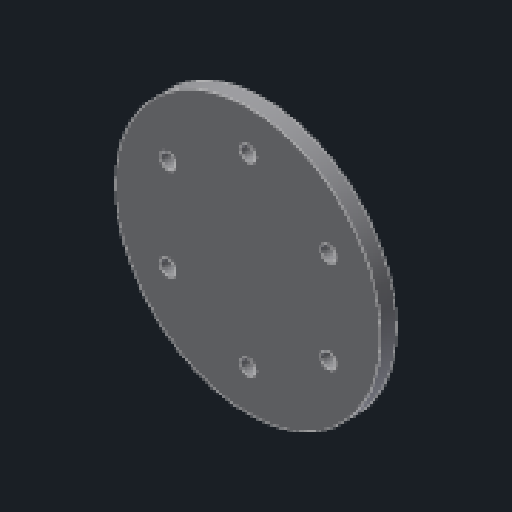
# Autodesk Inventor part: WheelSproketHub
Saved by Autodesk Inventor 2025.2 (Build 292293000, 293)
## iProperties
Created: 2025-10-03
Part Number: WheelSproketHub
Material: Generic
Document SubType Name: Sheet Metal
Designer: valer
Density: 1 g/cm^3
Appearance: Default
Sheet Metal Rule: Default
Author: valer
Autodesk Inventor part; units mm, degrees
ref_plane "YZ Plane" through (0, 0, 0) normal (1, 0, 0) x (0, 1, 0)
ref_plane "XZ Plane" through (0, 0, 0) normal (0, 1, 0) x (-1, 0, 0)
ref_plane "XY Plane" through (0, 0, 0) normal (0, 0, 1) x (1, 0, 0)
sketch "Base" plane through (0, 0, 0) normal (0, 0, 1) x (1, 0, 0)
  circle A0 centre (0, 0) radius 34.1376
  circle A1 centre (0, 23.8125) radius 1.9939 projected
  circle A2 centre (20.6222, 11.9063) radius 1.9939 projected
  circle A3 centre (20.6222, -11.9062) radius 1.9939 projected
  circle A4 centre (0, -23.8125) radius 1.9939 projected
  circle A5 centre (-20.6222, -11.9062) radius 1.9939 projected
  circle A6 centre (-20.6222, 11.9063) radius 1.9939 projected
  circle A7 centre (0, 0) radius 12.25
  dimension "d2" = 68.2752
  dimension "d9" = 24.5
  constraints: 2 centre point, 2 coincident
  measures "d2" diameter of A0
  measures "d9" diameter of A7
extrude "BaseFeature" add sketch "Base" along normal blind 4
equation "\"BendRadius\" = Thickness"
equation "\"BendReliefWidth\" = Thickness"
equation "\"BendReliefDepth\" = 0.5 * Thickness"
equation "\"CornerReliefSize\" = 4 * Thickness"
equation "\"MinimumRemnant\" = 2 * Thickness"
equation "\"TransitionRadius\" = BendRadius"
equation "\"JacobiRadiusSize\" = BendRadius"
equation "\"GapSize\" = Thickness"
equation "\"d6\" = Thickness"
equation "\"Thickness\" = 3.048"
body "Solid1"
